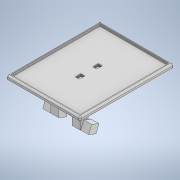
# Autodesk Inventor part: Piezatapa
Saved by Autodesk Inventor 2020 (Build 240168000, 168)
## iProperties
Created: 2019-10-30
Part Number: Piezatapa
Material: Genérico
Document SubType Name: Modeling
Designer: Daniel
Density: 1 g/cm^3
Appearance: Valor por defecto
Author: Daniel
Autodesk Inventor part; units mm, degrees
ref_plane "YZ Plane" through (0, 0, 0) normal (1, 0, 0) x (0, 1, 0)
ref_plane "XZ Plane" through (0, 0, 0) normal (0, 1, 0) x (-1, 0, 0)
ref_plane "XY Plane" through (0, 0, 0) normal (0, 0, 1) x (1, 0, 0)
sketch "Boceto1" plane through (0, 0, 0) normal (0, 1, 0) x (-1, 0, 0)
  line L0 (0, 0) -> (-93, 0)
  line L1 (-93, 0) -> (-93, -118)
  line L2 (-93, -118) -> (0, -118)
  line L3 (0, -118) -> (0, 0)
  dimension "d0" = 93
  dimension "d1" = 118
  constraints: 8 end point, 2 parallel, 1 horizontal, 1 perpendicular
  measures "d0" distance of L2.end L1.end
  measures "d1" distance of L1.end L0.end
extrude "Extrusión1" add sketch "Boceto1" along normal blind 6
shell "Vaciado1" thickness 3 removed faces 1 at (62, 6, -39.3333)
sketch "Boceto11" plane through (3, 3, -3) normal (0, 1, 0) x (1, 0, 0)
  line L0 (40, 70) -> (45, 70)
  line L1 (45, 70) -> (45, 63)
  line L2 (45, 63) -> (40, 63)
  line L3 (40, 63) -> (40, 70)
  line L4 (40, 48) -> (45, 48)
  line L5 (45, 48) -> (45, 41)
  line L6 (45, 41) -> (40, 41)
  line L7 (40, 41) -> (40, 48)
  point P0 (-3, -3)
  dimension "d33" = 5
  dimension "d34" = 7
  dimension "d35" = 5
  dimension "d36" = 7
  constraints: 16 end point, 4 parallel, 2 horizontal, 2 perpendicular, 1 point on line
  measures "d33" distance of L1.end L2.end
  measures "d34" distance of L0.end L1.end
  measures "d35" distance of L5.end L6.end
  measures "d36" distance of L4.end L5.end
extrude "Extrusión8" cut sketch "Boceto11" against normal blind 7
sketch "Boceto12" plane through (0, 0, 0) normal (0, -1, 0) x (1, 0, 0)
  line L0 (28, -28) -> (38, -28)
  line L1 (38, -28) -> (38, -38)
  line L2 (38, -38) -> (28, -38)
  line L3 (28, -38) -> (28, -28)
  line L4 (55, -38) -> (65, -38)
  line L5 (65, -38) -> (65, -28)
  line L6 (65, -28) -> (55, -28)
  line L7 (55, -28) -> (55, -38)
  point P0 (0, 0)
  dimension "d39" = 10
  dimension "d40" = 10
  dimension "d41" = 10
  dimension "d42" = 10
  constraints: 16 end point, 4 parallel, 2 horizontal, 2 perpendicular
  measures "d39" distance of L1.end L2.end
  measures "d40" distance of L0.end L1.end
  measures "d41" distance of L6.end L5.end
  measures "d42" distance of L5.end L4.end
extrude "Extrusión9" add sketch "Boceto12" along normal blind 40
sketch "Boceto13" plane through (28, 0, -38) normal (-1, 0, 0) x (0, 0, 1)
  line L0 (10, -40) -> (0, -40) projected
  line L1 (0, -40) -> (10, -35.9597)
  line L2 (10, 0) -> (10, -40) projected
  line L3 (0, -40) -> (10.7853, -40) construction
  point P0 (38, 0)
  dimension "d45" = 22
  constraints: 4 end point, 1 equal length, 1 horizontal, 1 point on line
  measures "d45" angle of L3 L1
extrude "Extrusión10" cut sketch "Boceto13" against normal blind 40
sketch "Boceto14" plane through (28, -35.9597, -28) normal (0, -0.9272, 0.3746) x (1, 0, 0)
  line L0 (0, 13.4708) -> (0, 0) projected
  line L1 (0, 0) -> (-10, 0)
  line L2 (-10, 0) -> (-10, -10)
  line L3 (-10, -10) -> (0, -10)
  line L4 (0, -10) -> (0, 0)
  line L5 (37, 0) -> (37, -10.7853) projected
  line L6 (37, -10.7853) -> (47, -10.7853)
  line L7 (47, -10.7853) -> (47, -0.7853)
  line L8 (47, -0.7853) -> (37, -0.7853)
  line L9 (37, -0.7853) -> (37, -10.7853)
  point P0 (-28, 39.4319)
  point P1 (37, -0.7853)
  dimension "d48" = 10
  dimension "d49" = 10
  dimension "d50" = 10
  dimension "d51" = 10
  constraints: 16 end point, 4 parallel, 2 horizontal, 2 perpendicular
  measures "d48" distance of L3.end L2.end
  measures "d49" distance of L2.end L1.end
  measures "d50" distance of L8.end L7.end
  measures "d51" distance of L7.end L6.end
extrude "Extrusión11" add sketch "Boceto14" against normal blind 10
fillet "Empalme1" radius 2 12 edges at (93, 6, -59) (93, 0, -59) (46.5, 0, -118) (46.5, 6, -118) (0, 6, -59) (0, 0, -59) (0, 3, -118) (93, 3, -118) (0, 3, 0) (46.5, 6, 0) (46.5, 0, 0) (93, 3, 0)
